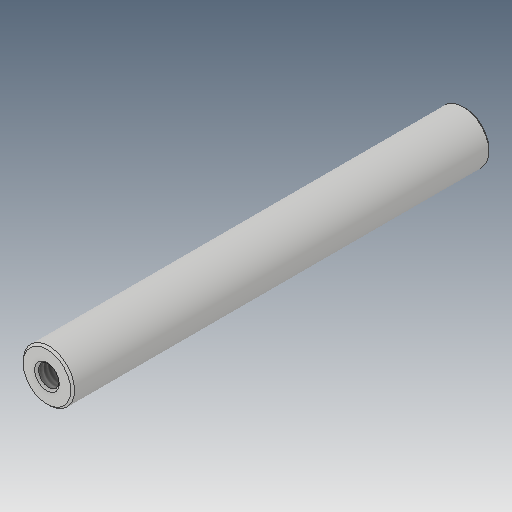
# Autodesk Inventor part: p8l65ALshaft
Saved by Autodesk Inventor 2019.4 (Build 234330000, 330)
## iProperties
Created: 2019-06-14
Part Number: p8l65ALshaft
Material: Generic
Document SubType Name: Modeling
Designer: AzLIer
Density: 1 g/cm^3
Appearance: Default
Mass: 2.7275 g
Surface Area: 23.6726 cm^2
Volume: 2.7275 cm^3
Author: AzLIer
Autodesk Inventor part; units mm, degrees
ref_plane "YZ Plane" through (0, 0, 0) normal (1, 0, 0) x (0, 1, 0)
ref_plane "XZ Plane" through (0, 0, 0) normal (0, 1, 0) x (-1, 0, 0)
ref_plane "XY Plane" through (0, 0, 0) normal (0, 0, 1) x (1, 0, 0)
sketch "スケッチ1" plane through (0, 0, 0) normal (0, 0, 1) x (1, 0, 0)
  circle A0 centre (0, 0) radius 4
  dimension "d0" = 8
  constraints: 1 centre point, 1 coincident
  measures "d0" diameter of A0
extrude "押し出し1" add sketch "スケッチ1" along normal blind 65
sketch "スケッチ2" plane through (0, 0, 65) normal (0, 0, 1) x (1, 0, 0)
  point P0 (0, 0)
hole "穴1" at (0, 0, 65) direction (0, 0, -1) diameter 3.242 end through all thread size "M4x0.7" class "6H" standard "ISO Metric profile"
chamfer "面取り1" distance 0.3 angle 45 4 edges at (-4, 0, 65) (0, 1.621, 65) (0, 1.621, 0) (-4, 0, 0)
